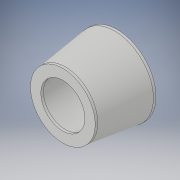
# Autodesk Inventor part: ecomake end part
Saved by Autodesk Inventor 2019 (Build 230136000, 136)
## iProperties
Created: 2019-10-20
Part Number: ecomake end part
Material: Generic
Document SubType Name: Modeling
Designer: Connor Duggan
Density: 1 g/cm^3
Appearance: Default
Mass: 421.153 g
Surface Area: 591.963 cm^2
Volume: 421.153 cm^3
Author: Connor Duggan
Autodesk Inventor part; units mm, degrees
ref_plane "YZ Plane" through (0, 0, 0) normal (1, 0, 0) x (0, 1, 0)
sketch "Sketch2" plane through (0, 0, 0) normal (0, 0, 1) x (1, 0, 0)
  circle A0 centre (0, 0) radius 19.05
  circle A1 centre (0, 0) radius 12.7
  dimension "d0" = 38.1
  dimension "d1" = 25.4
  constraints: 2 centre point, 2 coincident
  measures "d0" diameter of A0
  measures "d1" diameter of A1
ref_plane "Work Plane1" through (0, 0, 26.67) normal (0, 0, 1) x (1, 0, 0)
sketch "Sketch3" plane through (0, 0, 26.67) normal (0, 0, 1) x (1, 0, 0)
  circle A0 centre (0, 0) radius 15.875
  circle A1 centre (0, 0) radius 10.795
  dimension "d5" = 31.75
  dimension "d6" = 21.59
  constraints: 2 centre point, 2 coincident
  measures "d5" diameter of A0
  measures "d6" diameter of A1
extrude "Extrusion2" add sketch "Sketch3" against normal blind 1.27
extrude "Extrusion3" add sketch "Sketch2" along normal blind 1.27
sketch "Sketch4" plane through (0, 0, 26.67) normal (0, 0, 1) x (1, 0, 0)
  circle A0 centre (0, 0) radius 19.05 projected
  line L0 (0, 19.05) -> (0, 0) construction
  constraints: 2 end point, 1 vertical, 1 vertical alignment, 1 other
ref_plane "Work Plane2" through (0, 19.05, 26.67) normal (1, 0, 0) x (0, -1, 0)
sketch "Sketch5" plane through (0, 19.05, 26.67) normal (1, 0, 0) x (0, -1, 0)
  line L0 (34.925, 1.27) -> (3.175, 1.27)
  line L1 (0, 25.4) -> (38.1, 25.4)
  line L2 (3.175, 1.27) -> (0, 25.4)
  line L3 (8.255, 1.27) -> (29.845, 1.27)
  line L4 (31.75, 25.4) -> (6.35, 25.4)
  line L5 (6.35, 1.27) -> (6.35, 25.4)
  line L6 (6.35, 25.4) -> (0, 25.4)
  line L7 (8.255, 1.27) -> (3.175, 1.27)
  line L8 (19.05, -0.091501) -> (19.05, 9.410296) construction
  point P0 (19.05, 26.67)
  constraints: 10 end point, 2 vertical, 1 horizontal, 1 perpendicular
sketch "Sketch5 outline for Revolution1" plane through (0, 19.05, 26.67) normal (1, 0, 0) x (0, -1, 0)
  line L0 (0, 25.4) -> (3.175, 1.27)
  line L1 (6.35, 25.4) -> (0, 25.4)
  line L2 (8.255, 1.27) -> (6.35, 25.4)
  line L3 (3.175, 1.27) -> (8.255, 1.27)
revolve "Revolution1" add sketch "Sketch5 outline for Revolution1" angle 360 about axis through (0, 0, 26.761501) along (0, 0, -1)
body "Solid3"
